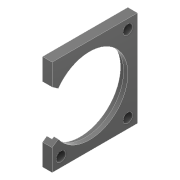
# Autodesk Inventor part: LargeLensHolderP2S1
Saved by Autodesk Inventor 2022 (Build 260153000, 153)
## iProperties
Created: 2021-12-05
Part Number: LargeLensHolderP2S1
Material: Acetal Resin, Black
Document SubType Name: Modeling
Designer: eganc
Density: 1.425 g/cm^3
Appearance: Smooth - Black
Author: eganc
Autodesk Inventor part; units mm, degrees
ref_plane "YZ Plane" through (0, 0, 0) normal (1, 0, 0) x (0, 1, 0)
ref_plane "XZ Plane" through (0, 0, 0) normal (0, 1, 0) x (-1, 0, 0)
ref_plane "XY Plane" through (0, 0, 0) normal (0, 0, 1) x (1, 0, 0)
sketch "Sketch1" plane through (0, 0, 0) normal (1, 0, 0) x (0, 1, 0)
  line L0 (-15, 15) -> (15, 15)
  line L1 (15, 15) -> (15, -15)
  line L2 (15, -15) -> (-15, -15)
  line L3 (-15, -15) -> (-15, 15)
  line L4 (-15, 15) -> (15, -15) construction
  line L5 (15, 15) -> (-15, -15) construction
  point P0 (0, 0)
  dimension "d0" = 30
  dimension "d1" = 30
  constraints: 12 end point, 2 midpoint, 2 parallel, 1 horizontal, 1 perpendicular
  measures "d0" distance of L1.end L2.end
  measures "d1" distance of L0.end L1.end
extrude "Extrusion1" add sketch "Sketch1" along normal blind 3
sketch "Sketch2" plane through (0, 0, 0) normal (1, 0, 0) x (0, 1, 0)
  circle A0 centre (0, 0) radius 12.7
  dimension "d4" = 25.4
  constraints: 1 centre point, 1 coincident
  measures "d4" diameter of A0
extrude "Extrusion2" cut sketch "Sketch2" along normal blind 1.614
sketch "Sketch3" plane through (0, 0, 0) normal (-1, 0, 0) x (0, 0, 1)
  circle A0 centre (0, 0) radius 12
  dimension "d7" = 24
  constraints: 1 centre point, 1 coincident
  measures "d7" diameter of A0
extrude "Extrusion3" cut sketch "Sketch3" against normal up to next
sketch "Sketch4" plane through (0, 0, 0) normal (0, 1, 0) x (-1, 0, 0)
  line L0 (-1.614, 12.7) -> (-1.614, -12.7) projected
  line L1 (-1.614, 0) -> (-1.614, -12.5586)
  line L2 (-2.2305, 0) -> (-1.614, 0)
  arc A0 (-2.2305, 0) -> (-1.614, -12.5586) centre (125.9995, 0) ccw
  point P0 (0, 0)
  dimension "d10" = 12.5586
  dimension "d11" = 256.46
  constraints: 4 end point, 2 horizontal, 2 point on circle, 2 point on line, 1 centre point, 1 midpoint
  measures "d10" distance of L1.start L1.end
  measures "d11" diameter of A0
revolve "Revolution1" cut sketch "Sketch4" angle 360 about axis through (2.2305, 0, 0) along (-1, 0, 0)
sketch "Sketch7" plane through (3, 0, 0) normal (1, 0, 0) x (0, 0, -1)
  circle A0 centre (12, 12) radius 1.5
  circle A1 centre (12, -12) radius 1.5
  circle A2 centre (-9, -12) radius 1.5
  line L0 (15, 15) -> (-15, 15) projected
  line L1 (15, -15) -> (15, 15) projected
  line L2 (-15, -15) -> (15, -15) projected
  line L3 (-15, 15) -> (-15, -15) projected
  point P0 (0, 0)
  dimension "d24" = 3
  dimension "d25" = 3
  dimension "d26" = 3
  dimension "d27" = 3
  dimension "d28" = 3
  dimension "d29" = 3
  dimension "d30" = 6
  constraints: 3 centre point, 2 equal radius
  measures "d24" distance from line of L0 A0.centre
  measures "d25" distance from line of L1 A0.centre
  measures "d26" diameter of A0
  measures "d27" distance from line of L1 A1.centre
  measures "d28" distance from line of L2 A1.centre
  measures "d29" distance from line of L2 A2.centre
  measures "d30" distance from line of L3 A2.centre
extrude "Extrusion6" cut sketch "Sketch7" against normal up to surface (3 mm away) contours A0 | A1 | A2
sketch "Sketch8" plane through (3, 0, 0) normal (1, 0, 0) x (0, 0, -1)
  line L0 (0, 0) -> (-15, 0) construction
  line L1 (-15, 15) -> (-15, -15) projected
  line L2 (0, 0) -> (-11.75, -8.2274)
  line L3 (-11.75, -8.2274) -> (-11.75, -15)
  line L4 (-15, -15) -> (15, -15) projected
  line L5 (-11.75, -15) -> (-15, -15)
  line L6 (-15, -15) -> (-15, 0)
  line L7 (-15, -15) -> (-15, 15)
  line L8 (0, 0) -> (-11.75, 8.2274)
  line L9 (-11.75, 8.2274) -> (-11.75, 15)
  line L10 (-15, 15) -> (15, 15)
  dimension "d33" = 3.25
  dimension "d34" = 35
  constraints: 18 end point, 5 symmetric about line, 2 point on line, 1 collinear, 1 midpoint, 1 vertical
  measures "d33" distance between parallel lines of L1 L3
  measures "d34" angle of L0 L2
extrude "Extrusion7" cut sketch "Sketch8" against normal up to surface (3 mm away)
body "Solid1"
